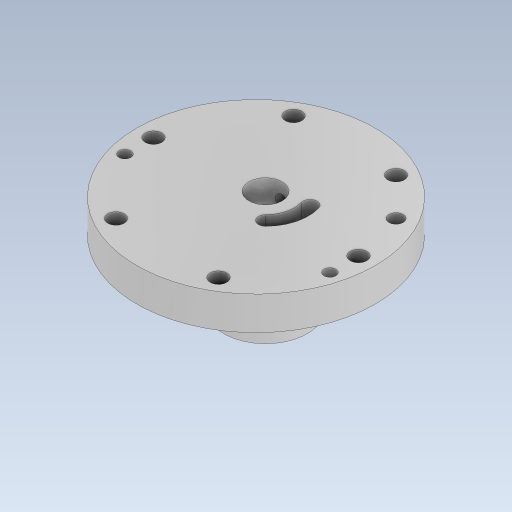
# Autodesk Inventor part: Pump-Motor-CW-Rotation:Casing 103
Saved by Autodesk Inventor 2024.2 (Build 282272000, 272)
## iProperties
Created: 2025-06-16
Material: Aluminum 6061
Document SubType Name: Modeling
Density: 2.7 g/cm^3
Appearance: Aluminum - Polished
Designer: cw
Author: cw
Autodesk Inventor part; units mm, degrees
note: some values were not read from the file. Chosen so that the rebuilt part matches the saved one: direction of "Hole5".
ref_plane "YZ Plane" through (0, 0, 0) normal (1, 0, 0) x (0, 1, 0)
sketch "Sketch1" plane through (0, 0, 0) normal (0, 0, 1) x (1, 0, 0)
  circle A0 centre (0, 0) radius 50
  dimension "d0" = 100
  constraints: 1 centre point, 1 coincident
  measures "d0" diameter of A0
extrude "Extrusion1" add sketch "Sketch1" along normal blind 14
sketch "Sketch2" plane through (0, 0, 0) normal (0, 0, -1) x (-1, 0, 0)
  circle A0 centre (0, 4) radius 23
  point P0 (0, 0)
  dimension "d3" = 4
  dimension "d4" = 46
  constraints: 1 centre point, 1 vertical alignment
  measures "d3" distance of A0.centre point (0, 0)
  measures "d4" diameter of A0
extrude "Extrusion2" add sketch "Sketch2" along normal blind 19
sketch "Sketch3" plane through (0, 0, 0) normal (0, 0, -1) x (-1, 0, 0)
  circle A0 centre (0, 4) radius 23 construction
  circle A1 centre (0, 4) radius 17.5
  point P0 (0, 0)
  dimension "d7" = 35
  constraints: 1 centre point, 1 coincident
  measures "d7" diameter of A1
extrude "Extrusion3" add sketch "Sketch3" along normal blind 29
sketch "Sketch4" plane through (0, 4, -29) normal (0, 0, -1) x (-1, 0, 0)
  circle A0 centre (0, 0) radius 17.5 construction
  point P0 (0, -4)
hole "Hole1" at (0, 4, -29) direction (0, 0, 1) diameter 14 end through all
sketch "Sketch5" plane through (0, 4, -29) normal (0, 0, -1) x (-1, 0, 0)
  circle A0 centre (0, 0) radius 17.5 construction
  point P0 (0, -4)
hole "Hole2" at (0, 4, -29) direction (0, 0, 1) diameter 28 depth 8
sketch "Sketch6" plane through (0, 0, 14) normal (0, 0, 1) x (1, 0, 0)
  circle A0 centre (0, 0) radius 43 construction
  point P0 (-43, 0)
  dimension "d24" = 86
  constraints: 1 coincident, 1 horizontal alignment, 2 other
hole "Hole3" at (-43, 0, 14) direction (0, 0, -1) diameter 7 end through all
pattern_circular "Circular Pattern1" count 6 over 360 about axis through (0, 0, 0) along (0, 0, 1) of "Hole3"
sketch "Sketch7" plane through (0, 0, 14) normal (0, 0, 1) x (1, 0, 0)
  circle A0 centre (-43, 0) radius 3.5 construction
  circle A1 centre (43, 0) radius 3.5 construction
  point P0 (0, 0)
  point P1 (-43, -12)
  point P2 (43, -12)
  dimension "d35" = 12
  constraints: 2 vertical alignment, 1 horizontal alignment
  measures "d35" distance of A1.centre point (43, -12)
hole "Hole4" at (-43, -12, 14) at (43, -12, 14) direction (0, 0, -1) diameter 5 depth 6 tip angle 118
sketch "Sketch8" plane through (0, 0, 14) normal (0, 0, 1) x (1, 0, 0)
  circle A0 centre (0, 4) radius 7 construction
  circle A1 centre (0, 0) radius 43 construction
  line L0 (-70, 0) -> (70, 0) construction
  line L1 (0, 0) -> (37.2391, 21.5) construction
  circle A2 centre (37.2391, 21.5) radius 3
  arc A3 (10.6066, -6.6066) -> (14.3713, 8.2973) centre (0, 4) ccw construction
  arc A4 (12.7279, -8.7279) -> (17.2455, 9.1567) centre (0, 4) ccw
  arc A5 (8.4853, -4.4853) -> (11.497, 7.4378) centre (0, 4) ccw
  arc A6 (8.4853, -4.4853) -> (12.7279, -8.7279) centre (10.6066, -6.6066) ccw
  arc A7 (17.2455, 9.1567) -> (11.497, 7.4378) centre (14.3713, 8.2973) ccw
  line L2 (0, 4) -> (15, 4) construction
  line L3 (0, 4) -> (10.6066, -6.6066) construction
  dimension "d43" = 86
  dimension "d44" = 30
  dimension "d45" = 6
  dimension "d46" = 15
  dimension "d48" = 45
  dimension "d49" = 6
  constraints: 11 point on circle, 6 centre point, 6 end point, 4 coincident, 4 tangent, 1 horizontal, 1 point on line, 3 other
  measures "d44" angle of L0 L1
  measures "d45" diameter of A2
  measures "d46" radius of A3
  measures "d48" angle of L3 L2
  measures "d49" radial gap between concentric circles of A4 A5
extrude "Extrusion4" cut sketch "Sketch8" against normal blind 7.5
ref_plane "Work Plane1" through (0, 0, 9) normal (0, 0, 1) x (1, 0, 0)
sketch "Sketch9" plane through (0, 0, 9) normal (0, 0, 1) x (1, 0, 0)
  circle A0 centre (37.2391, 21.5) radius 3 construction
  arc A1 (17.2455, 9.1567) -> (11.497, 7.4378) centre (14.3713, 8.2973) ccw construction
  line L0 (37.2391, 21.5) -> (14.3713, 8.2973)
  line L1 (14.3713, 8.2973) -> (13.1213, 10.4623)
  line L2 (13.1213, 10.4623) -> (35.9891, 23.6651)
  line L3 (35.9891, 23.6651) -> (37.2391, 21.5)
  point P0 (0, 0)
  dimension "d53" = 5
  constraints: 8 end point, 2 parallel, 1 perpendicular
  measures "d53" diameter of L2 L0
revolve "Revolution1" cut sketch "Sketch9" angle 360 about axis through (37.2391, 21.5, 9) along (-0.8660254, -0.5, 0)
ref_plane "Work Plane2" through (0, 50, 0) normal (0, 1, 0) x (-1, 0, 0)
sketch "Sketch10" plane through (0, 50, 0) normal (0, 1, 0) x (-1, 0, 0)
  line L0 (50, 14) -> (-50, 14) construction
  point P0 (0, 0)
  point P1 (0, 7)
  dimension "d55" = 7
  constraints: 1 vertical alignment
  measures "d55" distance from line of point (0, 7) L0
hole "Hole5" at (0, 50, 7) direction (0, -1, 0) diameter 4.917 end up to surface counterbore diameter 13.5 counterbore depth 1 thread size "M6x1" class "6H" standard "ISO Metric profile"
sketch "Sketch11" plane through (0, 4, -21) normal (0, 0, -1) x (-1, 0, 0)
  circle A0 centre (0, 0) radius 7 projected
  circle A1 centre (0, 0) radius 14 projected
  circle A2 centre (0, 0) radius 13
  dimension "d63" = 26
  constraints: 1 centre point, 1 coincident
  measures "d63" diameter of A2
extrude "Extrusion5" cut sketch "Sketch11" against normal blind 1 contours A2
sketch "Sketch12" plane through (0, 0, 0) normal (1, 0, 0) x (0, 1, 0)
  line L0 (49, 13.75) -> (49, 9.4585) projected
  line L1 (49, 9.4585) -> (11, 9.4585) projected
  line L2 (11, 9.4585) -> (11, 14) projected
  line L3 (11, 14) -> (50, 14) projected
  line L4 (50, 14) -> (50, 13.75) projected
  line L5 (50, 13.75) -> (49, 13.75) projected
  line L6 (27, 0) -> (27, -19) projected
  line L7 (27, -19) -> (21.5, -19) projected
  line L8 (21.5, -19) -> (21.5, -29) projected
  line L9 (21.5, -29) -> (18, -29) projected
  line L10 (18, -29) -> (18, -21) projected
  line L11 (18, -21) -> (17, -21) projected
  line L12 (17, -21) -> (17, -20) projected
  line L13 (17, -20) -> (11, -20) projected
  line L14 (11, -20) -> (11, 4.5415) projected
  line L15 (11, 4.5415) -> (49, 4.5415) projected
  line L16 (49, 4.5415) -> (49, 0.25) projected
  line L17 (49, 0.25) -> (50, 0.25) projected
  line L18 (50, 0.25) -> (50, 0) projected
  line L19 (50, 0) -> (27, 0) projected
  line L20 (-50, 0) -> (-50, 14) projected
  line L21 (-50, 14) -> (-3, 14) projected
  line L22 (-3, 14) -> (-3, -20) projected
  line L23 (-3, -20) -> (-9, -20) projected
  line L24 (-9, -20) -> (-9, -21) projected
  line L25 (-9, -21) -> (-10, -21) projected
  line L26 (-10, -21) -> (-10, -29) projected
  line L27 (-10, -29) -> (-13.5, -29) projected
  line L28 (-13.5, -29) -> (-13.5, -19) projected
  line L29 (-13.5, -19) -> (-19, -19) projected
  line L30 (-19, -19) -> (-19, 0) projected
  line L31 (-19, 0) -> (-50, 0) projected
  line L32 (-3, 14) -> (-3, -20) projected
  line L33 (-3, -2.3) -> (-8, -2.3)
  line L34 (-8, -2.3) -> (-8, -20)
  line L35 (-8, -20) -> (-3, -20)
  line L36 (-3, 14) -> (11, 14) projected
  line L37 (4, 14) -> (4, -29)
  line L38 (-8, -17.5) -> (-8.6, -17.5)
  line L39 (-8.6, -17.5) -> (-8.6, -16.2)
  line L40 (-8.6, -16.2) -> (-8, -16.2)
  point P0 (0, 0)
  dimension "d70" = 24
  dimension "d72" = 1.3
  dimension "d73" = 25.2
  dimension "d74" = 3.5
  dimension "d75" = 15.2
  constraints: 14 end point, 6 perpendicular, 5 point on line, 1 collinear, 1 midpoint, 1 vertical
  measures "d70" diameter of L34 L37
  measures "d72" distance between parallel lines of L40 L38
  measures "d73" diameter of L39 L37
  measures "d74" distance between parallel lines of L38 L25
  measures "d75" distance between parallel lines of L33 L38
revolve "Revolution2" cut sketch "Sketch12" angle 360 about axis through (0, 4, 14) along (0, 0, -1) contours L22 L23 L34 L33 | L34 L38 L39 L40
body "Solid1"
